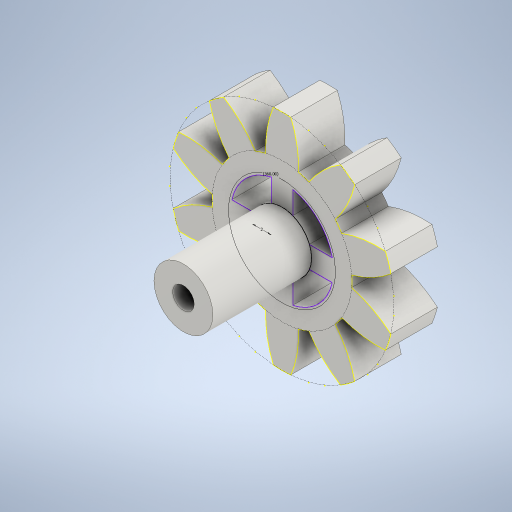
# Autodesk Inventor part: Spur Gear1
Saved by Autodesk Inventor 2023 (Build 270158000, 158)
## iProperties
CustomPartVersion: 1
Created: 2022-11-24
Part Number: Spur Gear1
Material: Steel
Document SubType Name: Modeling
Designer: shrey
Categories: <?xml version="1.0" encoding="UTF-16"?> <MemberInstance><Categories><FamilyTemplate><FamilyTemplateParameter ValueType="xs:double" Id="1" ObjectReferenceKey="da_z" ObjectType="kUserParameterObject"/><FamilyTemplateParameter ValueType="xs:double" Id="2" ObjectReferenceKey="da_b" ObjectType="kUserParameterObject"/><FamilyTemplateParameter ValueType="xs:double" Id="3" ObjectReferenceKey="da_beta" ObjectType="kUserParameterObject"/><FamilyTemplateParameter ValueType="xs:double" Id="4" ObjectReferenceKey="da_da" ObjectType="kUserParameterObject"/><FamilyTemplateParameter ValueType="xs:double" Id="5" ObjectReferenceKey="da_aw" ObjectType="kUserParameterObject"/><FamilyTemplateParameter ValueType="xs:string" Id="6" ObjectReferenceKey="EAIAABAAAACIAQAAAAAAAIAAAAAAAAAA" ObjectType="83910656" SubObjectId="SurfaceGeometry"/></FamilyTemplate><ParamToTemplateMap><ParamToTemplate CategoryParameter="//CategoryParameter[@InternalName='046C89C9-8512-4d59-83FE-43B91F4F132A']" TemplateParameter="1"/><ParamToTemplate CategoryParameter="//CategoryParameter[@InternalName='2552DF32-E462-4b46-AEBF-C6C7768E72AC']" TemplateParameter="2"/><ParamToTemplate CategoryParameter="//CategoryParameter[@InternalName='C9EE641D-15FC-4fae-A226-E94C4372FDD7']" TemplateParameter="3"/><ParamToTemplate><ParamToTemplate CategoryParameter="//CategoryParameter[@InternalName='00B6519A-459B-49c7-AD84-2E56D39A5744']" ConstantValue="0.000000"/></ParamToTemplate><ParamToTemplate><ParamToTemplate CategoryParameter="//CategoryParameter[@InternalName='04B31F0E-C7A6-4894-AA32-9629BEFACF47']" ConstantValue="1.000000"/></ParamToTemplate><ParamToTemplate><ParamToTemplate CategoryParameter="//CategoryParameter[@InternalName='43CBEC2E-7847-49e7-A936-2F7889FCB2D9']" ConstantValue="0.250000"/></ParamToTemplate><ParamToTemplate><ParamToTemplate CategoryParameter="//CategoryParameter[@InternalName='B1EFC894-105D-4ebd-86BF-FA20ED196853']" ConstantValue="0.350000"/></ParamToTemplate><ParamToTemplate><ParamToTemplate CategoryParameter="//CategoryParameter[@InternalName='51175063-3D10-4879-93E8-6246FE8B403D']" ConstantValue="2060000000.000000"/></ParamToTemplate><ParamToTemplate><ParamToTemplate CategoryParameter="//CategoryParameter[@InternalName='A3A52E27-4454-46a9-B0BD-C932399B70AF']" ConstantValue="0.300000"/></ParamToTemplate><ParamToTemplate><ParamToTemplate CategoryParameter="//CategoryParameter[@InternalName='91B76062-C214-41d9-B1B9-14D2AB99603D']" ConstantValue="0.200000"/></ParamToTemplate><ParamToTemplate><ParamToTemplate CategoryParameter="//CategoryParameter[@InternalName='374E806E-8B8A-4dda-A9AA-1039D6500AD2']" ConstantValue="5.000000"/></ParamToTemplate><ParamToTemplate><ParamToTemplate CategoryParameter="//CategoryParameter[@InternalName='2D373A89-B862-43d6-8D0B-0CBF12AB9F6C']" ConstantValue="0.349066"/></ParamToTemplate><ParamToTemplate CategoryParameter="//CategoryParameter[@InternalName='37777632-D6A2-4fac-9D53-DB8ACD95C989']" TemplateParameter="4"/><ParamToTemplate CategoryParameter="//CategoryParameter[@InternalName='FD1017F1-B727-4f7e-9707-0F86F1FF9423']" TemplateParameter="5"/><ParamToTemplate><ParamToTemplate CategoryParameter="//CategoryParameter[@InternalName='9E1B4470-B2D3-4ff1-B813-535BB4CDF51A']" ConstantValue="3520000.000000"/></ParamToTemplate><ParamToTemplate><ParamToTemplate CategoryParameter="//CategoryParameter[@InternalName='F8452263-BFF6-458c-9FB1-07C4B99E95CD']" ConstantValue="11400000.000000"/></ParamToTemplate><ParamToTemplate><ParamToTemplate CategoryParameter="//CategoryParameter[@InternalName='3E3BB259-FD49-497f-8171-6EBC954A3479']" ConstantValue="2.000000"/></ParamToTemplate><ParamToTemplate CategoryParameter="//CategoryParameter[@InternalName='27C3BAF2-7550-4e4b-AE2C-0DB134B7D9B7']" TemplateParameter="6"/></ParamToTemplateMap><Category DisplayName="Gear" InternalName="DC85795E-93AB-48d5-8EEE-5A27447B64BD" Mnemonic="Gear"><CategoryParameter DisplayName="z" InternalName="046C89C9-8512-4d59-83FE-43B91F4F132A" Mnemonic="z"/><CategoryParameter DisplayName="b" InternalName="2552DF32-E462-4b46-AEBF-C6C7768E72AC" Mnemonic="b"/><CategoryParameter DisplayName="||b|" InternalName="C9EE641D-15FC-4fae-A226-E94C4372FDD7" Mnemonic="beta"/><CategoryParameter DisplayName="x" InternalName="00B6519A-459B-49c7-AD84-2E56D39A5744" Mnemonic="x"/><CategoryParameter DisplayName="a*" InternalName="04B31F0E-C7A6-4894-AA32-9629BEFACF47" Mnemonic="a"/><CategoryParameter DisplayName="c*" InternalName="43CBEC2E-7847-49e7-A936-2F7889FCB2D9" Mnemonic="c"/><CategoryParameter DisplayName="r|.f|*" InternalName="B1EFC894-105D-4ebd-86BF-FA20ED196853" Mnemonic="rf"/><CategoryParameter DisplayName="E" InternalName="51175063-3D10-4879-93E8-6246FE8B403D" Mnemonic="E"/><CategoryParameter DisplayName="||m|" InternalName="A3A52E27-4454-46a9-B0BD-C932399B70AF" Mnemonic="mi"/><Category DisplayName="SpurGear" InternalName="26C5A22E-A91E-4dfd-A3B3-23CCAFAE1764" Mnemonic="SpurGear"><CategoryParameter DisplayName="m" InternalName="91B76062-C214-41d9-B1B9-14D2AB99603D" Mnemonic="m"/><CategoryParameter DisplayName="P" InternalName="374E806E-8B8A-4dda-A9AA-1039D6500AD2" Mnemonic="PP"/><CategoryParameter DisplayName="||a|" InternalName="2D373A89-B862-43d6-8D0B-0CBF12AB9F6C" Mnemonic="alpha"/><CategoryParameter DisplayName="d|.a|" InternalName="37777632-D6A2-4fac-9D53-DB8ACD95C989" Mnemonic="da"/><CategoryParameter DisplayName="a|.w|" InternalName="FD1017F1-B727-4f7e-9707-0F86F1FF9423" Mnemonic="aw"/><CategoryParameter DisplayName="||s||.Flim|" InternalName="9E1B4470-B2D3-4ff1-B813-535BB4CDF51A" Mnemonic="sFlim"/><CategoryParameter DisplayName="||s||.Hlim|" InternalName="F8452263-BFF6-458c-9FB1-07C4B99E95CD" Mnemonic="sHlim"/><CategoryParameter DisplayName="type" InternalName="3E3BB259-FD49-497f-8171-6EBC954A3479" Mnemonic="type"/><CategoryParameter DisplayName="PitchDiameter" InternalName="27C3BAF2-7550-4e4b-AE2C-0DB134B7D9B7" Mnemonic="IDS_PITCHDIAM"/></Category></Category></Categories></MemberInstance>
Density: 1 g/cm^3
Appearance: Steel
Author: shrey
Autodesk Inventor part; units mm, degrees
sketch "Sketch1" plane through (0, 0, 0) normal (0, 0, 1) x (1, 0, 0)
  circle A0 centre (0, 0) radius 12
  circle A1 centre (0, 0) radius 1.16
  dimension "d0" = 24
  dimension "d49" = 2.32
  constraints: 2 centre point, 1 coincident
  measures "d0" diameter of A0
  measures "d49" diameter of A1
extrude "Extrusion1" add sketch "Sketch1" along normal blind 5 contours A0 | A1
ref_plane "Work Plane2" through (0, 0, 2.5) normal (0, 0, 1) x (1, 0, 0)
sketch "Sketch2" plane through (0, 0, 0) normal (0, 0, -1) x (-1, 0, 0)
  circle A0 centre (0, 0) radius 12 projected
  circle A1 centre (0, 0) radius 10
  dimension "d3" = 20
  constraints: 1 centre point, 1 coincident
  measures "d3" diameter of A1
surface extrude "Pitch Diameter" sketch "Sketch2" against normal through all shown no curves A1
ref_plane "Work Plane8" through (0, 0, 0) normal (0.9510565, 0.309017, 0) x (0, 0, 1)
ref_plane "Work Plane9" through (0, 0, 0) normal (1, 0, 0) x (0, 1, 0)
spur gear teeth "Spur Gear" teeth 10 pitch diameter 20 tip diameter 24 root diameter 15 face width 5 start plane through (0, 0, 0) normal (0, 0, -1) x (-1, 0, 0)
extrude "Extrusion2" cut sketch "Sketch1" along normal blind 5 contours A1
sketch "Sketch4" plane through (0, 0, 5) normal (0, 0, 1) x (1, 0, 0)
  circle A0 centre (0, 0) radius 1.16 projected
  arc A1 (-7.7934, 9.1249) -> (-5.703, 4.8709) centre (2.8495, 11.714) ccw projected
  arc A2 (-5.703, 4.8709) -> (-6.3948, 3.9187) centre (0, 0) ccw projected
  arc A3 (-6.3948, 3.9187) -> (-11.0866, 4.5922) centre (-10.2601, -6.3299) ccw projected
  arc A4 (-11.0866, 4.5922) -> (-11.6684, 2.8013) centre (0, 0) ccw projected
  arc A5 (-11.6684, 2.8013) -> (-7.4769, 0.5884) centre (-4.58, 11.1517) ccw projected
  arc A6 (-7.4769, 0.5884) -> (-7.4769, -0.5884) centre (0, 0) ccw projected
  arc A7 (-7.4769, -0.5884) -> (-11.6684, -2.8013) centre (-4.58, -11.1517) ccw projected
  arc A8 (-11.6684, -2.8013) -> (-11.0866, -4.5922) centre (0, 0) ccw projected
  arc A9 (-11.0866, -4.5922) -> (-6.3948, -3.9187) centre (-10.2601, 6.3299) ccw projected
  arc A10 (-6.3948, -3.9187) -> (-5.703, -4.8709) centre (0, 0) ccw projected
  arc A11 (-5.703, -4.8709) -> (-7.7934, -9.1249) centre (2.8495, -11.714) ccw projected
  arc A12 (-7.7934, -9.1249) -> (-6.27, -10.2317) centre (0, 0) ccw projected
  arc A13 (-6.27, -10.2317) -> (-2.8701, -6.9291) centre (-12.0212, -0.9098) ccw projected
  arc A14 (-2.8701, -6.9291) -> (-1.7508, -7.2928) centre (0, 0) ccw projected
  arc A15 (-1.7508, -7.2928) -> (-0.9415, -11.963) centre (9.1906, -7.8019) ccw projected
  arc A16 (-0.9415, -11.963) -> (0.9415, -11.963) centre (0, 0) ccw projected
  arc A17 (0.9415, -11.963) -> (1.7508, -7.2928) centre (-9.1906, -7.8019) ccw projected
  arc A18 (1.7508, -7.2928) -> (2.8701, -6.9291) centre (0, 0) ccw projected
  arc A19 (2.8701, -6.9291) -> (6.27, -10.2317) centre (12.0212, -0.9098) ccw projected
  arc A20 (6.27, -10.2317) -> (7.7934, -9.1249) centre (0, 0) ccw projected
  arc A21 (7.7934, -9.1249) -> (5.703, -4.8709) centre (-2.8495, -11.714) ccw projected
  arc A22 (5.703, -4.8709) -> (6.3948, -3.9187) centre (0, 0) ccw projected
  arc A23 (6.3948, -3.9187) -> (11.0866, -4.5922) centre (10.2601, 6.3299) ccw projected
  arc A24 (11.0866, -4.5922) -> (11.6684, -2.8013) centre (0, 0) ccw projected
  arc A25 (11.6684, -2.8013) -> (7.4769, -0.5884) centre (4.58, -11.1517) ccw projected
  arc A26 (7.4769, -0.5884) -> (7.4769, 0.5884) centre (0, 0) ccw projected
  arc A27 (7.4769, 0.5884) -> (11.6684, 2.8013) centre (4.58, 11.1517) ccw projected
  arc A28 (11.6684, 2.8013) -> (11.0866, 4.5922) centre (0, 0) ccw projected
  arc A29 (11.0866, 4.5922) -> (6.3948, 3.9187) centre (10.2601, -6.3299) ccw projected
  arc A30 (6.3948, 3.9187) -> (5.703, 4.8709) centre (0, 0) ccw projected
  arc A31 (5.703, 4.8709) -> (7.7934, 9.1249) centre (-2.8495, 11.714) ccw projected
  arc A32 (7.7934, 9.1249) -> (6.27, 10.2317) centre (0, 0) ccw projected
  arc A33 (6.27, 10.2317) -> (2.8701, 6.9291) centre (12.0212, 0.9098) ccw projected
  arc A34 (2.8701, 6.9291) -> (1.7508, 7.2928) centre (0, 0) ccw projected
  arc A35 (1.7508, 7.2928) -> (0.9415, 11.963) centre (-9.1906, 7.8019) ccw projected
  arc A36 (0.9415, 11.963) -> (-0.9415, 11.963) centre (0, 0) ccw projected
  arc A37 (-0.9415, 11.963) -> (-1.7508, 7.2928) centre (9.1906, 7.8019) ccw projected
  arc A38 (-1.7508, 7.2928) -> (-2.8701, 6.9291) centre (0, 0) ccw projected
  arc A39 (-2.8701, 6.9291) -> (-6.27, 10.2317) centre (-12.0212, 0.9098) ccw projected
  arc A40 (-6.27, 10.2317) -> (-7.7934, 9.1249) centre (0, 0) ccw projected
  arc A41 (1.7508, 7.2928) -> (0.9415, 11.963) centre (-9.1906, 7.8019) ccw construction
  circle A42 centre (0, 0) radius 12 construction
  circle A43 centre (0, 0) radius 1.16 construction
  circle A44 centre (0, 0) radius 7.5 construction
  circle A45 centre (0, 0) radius 3.16
  line L0 (-1.16, 5.3763) -> (-1.16, 2.9394)
  line L1 (1.16, 2.9394) -> (1.16, 5.3763)
  line L2 (-5.3763, -1.16) -> (-2.9394, -1.16)
  line L3 (-2.9394, 1.16) -> (-5.3763, 1.16)
  line L4 (1.16, -5.3763) -> (1.16, -2.9394)
  line L5 (-1.16, -2.9394) -> (-1.16, -5.3763)
  line L6 (5.3763, 1.16) -> (2.9394, 1.16)
  line L7 (2.9394, -1.16) -> (5.3763, -1.16)
  arc A46 (-1.16, 5.3763) -> (-5.3763, 1.16) centre (0, 0) ccw
  arc A47 (5.3763, 1.16) -> (1.16, 5.3763) centre (0, 0) ccw
  arc A48 (-5.3763, -1.16) -> (-1.16, -5.3763) centre (0, 0) ccw
  arc A49 (1.16, -5.3763) -> (5.3763, -1.16) centre (0, 0) ccw
  dimension "d62" = 2
  dimension "d66" = 360
  constraints: 16 end point, 10 point on circle, 6 centre point, 2 coincident, 1 concentric, 1 tangent, 28 other
  measures "d62" radial gap between concentric circles of A0 A45
extrude "Extrusion5" cut sketch "Sketch4" against normal through all contours A45 L1 A47 L6 | L7 A49 L4 A45 | A45 L3 A46 L0 | L5 A48 L2 A45
extrude "Extrusion6" add sketch "Sketch4" along normal blind 10.56 contours A45
equation "\"d0\" = da_da"
equation "\"d3\" = da_d"
equation "\"da_da\" = 24"
equation "\"da_d\" = 20"
body "Solid1"
body "Srf1"
